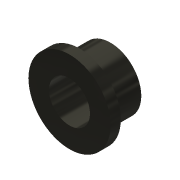
# Autodesk Inventor part: Flange Sleve Bearing .25.375
Saved by Autodesk Inventor 2014 (Build 180170000, 170)
## iProperties
Created: 2014-07-18
Part Number: Flange Sleve Bearing .25.375
Material: Generic
Document SubType Name: Modeling
Designer: Owner
Density: 1 g/cm^3
Appearance: Gunmetal
Author: Owner
Autodesk Inventor part; units mm, degrees
ref_plane "YZ Plane" through (0, 0, 0) normal (1, 0, 0) x (0, 1, 0)
ref_plane "XZ Plane" through (0, 0, 0) normal (0, 1, 0) x (-1, 0, 0)
ref_plane "XY Plane" through (0, 0, 0) normal (0, 0, 1) x (1, 0, 0)
sketch "Sketch1" plane through (0, 0, 0) normal (0, 0, 1) x (1, 0, 0)
  circle A0 centre (0, 0) radius 3.175
  circle A1 centre (0, 0) radius 4.7625
  circle A2 centre (0, 0) radius 6.35
  dimension "d2" = 6.35
  dimension "d3" = 9.525
  dimension "d4" = 12.7
  constraints: 3 centre point, 3 coincident
  measures "d2" diameter of A0
  measures "d3" diameter of A1
  measures "d4" diameter of A2
extrude "Extrusion1" add sketch "Sketch1" against normal blind 6.35 contours A1
extrude "Extrusion2" add sketch "Sketch1" against normal blind 1.5875 contours A2
body "Solid1"
